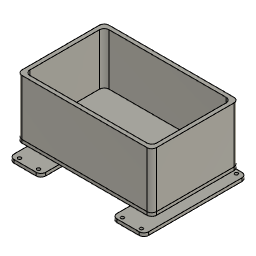
PondPumpFixture v5 (Autodesk Fusion 360 design; units mm, degrees)
Autodesk Fusion 360 part; units mm, degrees
sketch "Sketch1" plane through (0, 0, 0) normal (0, 0, 1) x (1, 0, 0)
  line L0 (0, 0) -> (160, 0)
  line L1 (160, 0) -> (160, 100)
  line L2 (160, 100) -> (0, 100)
  line L3 (0, 100) -> (0, 0)
  line L4 (0, 50) -> (160, 50) construction
  line L5 (125, 100) -> (125, 0) construction
  circle A0 centre (125, 84.5) radius 2
  circle A1 centre (125, 15.5) radius 2
  circle A2 centre (15, 85) radius 8
  circle A3 centre (15, 85) radius 4.75
  line L6 (-5, -5) -> (165, -5)
  line L7 (165, -5) -> (165, 105)
  line L8 (165, 105) -> (-5, 105)
  line L9 (-5, 105) -> (-5, -5)
  circle A4 centre (15, 15) radius 8
  circle A5 centre (15, 15) radius 4.75
  circle A6 centre (145, 85) radius 8
  circle A7 centre (145, 85) radius 4.75
  circle A8 centre (145, 15) radius 8
  circle A9 centre (145, 15) radius 4.75
  line L10 (-5, 105) -> (35, 105)
  line L11 (35, 105) -> (35, 115)
  line L12 (35, 115) -> (-5, 115)
  line L13 (-5, 115) -> (-5, 105)
  line L14 (15, 115) -> (15, -15) construction
  line L15 (-5, -5) -> (35, -5)
  line L16 (35, -5) -> (35, -15)
  line L17 (35, -15) -> (-5, -15)
  line L18 (-5, -15) -> (-5, -5)
  line L19 (-5, 110) -> (35, 110) construction
  circle A10 centre (3, 110) radius 2
  circle A11 centre (27, 110) radius 2
  line L20 (-5, -10) -> (35, -10) construction
  circle A12 centre (3, -10) radius 2
  circle A13 centre (27, -10) radius 2
  line L21 (35, -5) -> (35, 105)
  line L22 (165, 105) -> (125, 105)
  line L23 (125, 105) -> (125, 115)
  line L24 (125, 115) -> (165, 115)
  line L25 (165, 115) -> (165, 105)
  line L26 (165, -5) -> (125, -5)
  line L27 (125, -5) -> (125, -15)
  line L28 (125, -15) -> (165, -15)
  line L29 (165, -15) -> (165, -5)
  line L30 (125, -5) -> (125, 105)
  line L31 (145, 115) -> (145, -15) construction
  line L32 (125, 110) -> (165, 110) construction
  line L33 (125, -10) -> (165, -10) construction
  circle A14 centre (133, 110) radius 2
  circle A15 centre (157, 110) radius 2
  circle A16 centre (133, -10) radius 2
  circle A17 centre (157, -10) radius 2
  dimension "d1" = 160
  dimension "d2" = 100
  dimension "d3" = 4
  dimension "d4" = 4
  dimension "d5" = 34.5
  dimension "d6" = 34.5
  dimension "d7" = 35
  dimension "d8" = 16
  dimension "d9" = 9.5
  dimension "d12" = 5
  dimension "d13" = 16
  dimension "d14" = 9.5
  dimension "d16" = 15
  dimension "d17" = 16
  dimension "d18" = 9.5
  dimension "d19" = 16
  dimension "d20" = 9.5
  dimension "d22" = 15
  dimension "d23" = 15
  dimension "d25" = 40
  dimension "d26" = 10
  dimension "d28" = 40
  dimension "d29" = 10
  dimension "d30" = 15
  dimension "d31" = 4
  dimension "d32" = 4
  dimension "d33" = 8
  dimension "d34" = 8
  dimension "d35" = 4
  dimension "d36" = 4
  dimension "d37" = 8
  dimension "d38" = 8
  dimension "d39" = 40
  dimension "d40" = 10
  dimension "d41" = 40
  dimension "d42" = 10
  dimension "d43" = 4
  dimension "d44" = 4
  dimension "d45" = 8
  dimension "d46" = 8
  dimension "d47" = 4
  dimension "d48" = 4
  dimension "d49" = 8
  dimension "d50" = 8
  constraint horizontal L0
  constraint vertical L1
  constraint horizontal L2
  constraint vertical L3
  constraint coincident L0.start L3.end
  constraint midpoint L3 L4.start
  constraint midpoint L1 L4.end
  constraint coincident L2 L5.start
  constraint coincident L0 L5.end
  constraint perpendicular L0 L5
  constraint coincident L5 A0.centre
  constraint coincident L5 A1.centre
  constraint concentric A2 A3
  constraint concentric A4 A5
  constraint concentric A6 A7
  constraint concentric A8 A9
  constraint horizontal L10
  constraint vertical L11
  constraint horizontal L12
  constraint vertical L13
  constraint midpoint L12 L14.start
  constraint perpendicular L6 L14
  constraint horizontal L15
  constraint vertical L16
  constraint horizontal L17
  constraint vertical L18
  constraint midpoint L14.end L17
  constraint coincident A4.centre L14
  constraint coincident A2.centre L14
  constraint midpoint L13 L19.start
  constraint midpoint L11 L19.end
  constraint coincident L19 A10.centre
  constraint coincident L19 A11.centre
  constraint midpoint L18 L20.start
  constraint midpoint L16 L20.end
  constraint coincident L20 A12.centre
  constraint coincident L20 A13.centre
  constraint horizontal L22
  constraint vertical L23
  constraint horizontal L24
  constraint vertical L25
  constraint horizontal L26
  constraint vertical L27
  constraint horizontal L28
  constraint vertical L29
  constraint midpoint L24 L31.start
  constraint midpoint L28 L31.end
  constraint coincident A6.centre L31
  constraint coincident A8.centre L31
  constraint midpoint L23 L32.start
  constraint midpoint L25 L32.end
  constraint midpoint L27 L33.start
  constraint midpoint L29 L33.end
  constraint coincident L32 A14.centre
  constraint coincident L32 A15.centre
  constraint coincident L33 A16.centre
  constraint coincident L33 A17.centre
  measures "d1" distance of L0.start L0.end
  measures "d2" distance of L0.start L2.end
  measures "d3" diameter of A0
  measures "d4" diameter of A1
  measures "d5" distance of L4 A0.centre
  measures "d6" distance of L4 A1.centre
  measures "d7" distance of L1 L5
  measures "d8" diameter of A2
  measures "d9" diameter of A3
  measures "d13" diameter of A4
  measures "d14" diameter of A5
  measures "d16" distance of L0 A4.centre
  measures "d17" diameter of A6
  measures "d18" diameter of A7
  measures "d19" diameter of A8
  measures "d20" diameter of A9
  measures "d22" distance of L0 A8.centre
  measures "d23" distance of L2 A6.centre
  measures "d25" distance of L8.end L10.end
  measures "d26" distance of L8.end L12.end
  measures "d28" distance of L6.start L15.end
  measures "d29" distance of L6.start L17.end
  measures "d30" distance of L2 A2.centre
  measures "d31" diameter of A10
  measures "d32" diameter of A11
  measures "d33" distance of L19.end A11.centre
  measures "d34" distance of L13 A10.centre
  measures "d35" diameter of A12
  measures "d36" diameter of A13
  measures "d37" distance of L20.start A12.centre
  measures "d38" distance of L20.end A13.centre
  measures "d39" distance of L7.end L22.end
  measures "d40" distance of L7.end L24.end
  measures "d41" distance of L6.end L26.end
  measures "d42" distance of L6.end L28.end
  measures "d43" diameter of A14
  measures "d44" diameter of A15
  measures "d45" distance of L32.start A14.centre
  measures "d46" distance of L32.end A15.centre
  measures "d47" diameter of A16
  measures "d48" diameter of A17
  measures "d49" distance of L33.start A16.centre
  measures "d50" distance of L33.end A17.centre
extrude "Extrude1" add sketch "Sketch1" along normal blind 5 contours L0 L2 L3 L21 | L0 L2 L3 L6 L8 L9 L10 L15 L21 | L0 L2 A0 A1 L21 L30 | L0 L6 L21 L30 | L0 L1 L2 A0 A1 L30 | L0 L1 L2 L6 L7 L8 L22 L26 L30 | L2 L8 L21 L30 | A2 | A3 | A4 | A5 | A6 | A7 | A8 | A9 makes body 1
extrude "Extrude2" add sketch "Sketch1" along normal blind 70 contours L0 L2 L3 L6 L8 L9 L10 L15 L21 | L0 L6 L21 L30 | L0 L1 L2 L6 L7 L8 L22 L26 L30 | L2 L8 L21 L30 bodies 1
extrude "Extrude3" add sketch "Sketch1" against normal blind 4 separate body contours L0 L2 L3 L21 | L0 L2 L3 L6 L8 L9 L10 L15 L21 | L0 L2 A0 A1 L21 L30 | L0 L6 L21 L30 | L0 L1 L2 A0 A1 L30 | L0 L1 L2 L6 L7 L8 L22 L26 L30 | L2 L8 L21 L30 | A1 L30 | A1 L30 | A0 L30 | A0 L30 makes body 2
extrude "Extrude4" add sketch "Sketch1" against normal blind 2 from surface at -2 contours A2 | A4 | A6 | A8 bodies 2
extrude "Extrude5" add sketch "Sketch1" against normal blind 4 from surface at -17 separate body contours L0 L2 L3 L21 | L0 L2 L3 L6 L8 L9 L10 L15 L21 | L0 L1 L2 A0 A1 L30 | L0 L1 L2 L6 L7 L8 L22 L26 L30 | L6 L15 L16 L17 L18 | L6 L26 L27 L28 L29 | A1 L30 | L8 L10 L11 L12 L13 | A0 L30 | L8 L22 L23 L24 L25 picked at (125.6397, 15.3122) picked at (125.6397, 84.3122) makes body 3 at (-0.9702, 38.7308, -17) makes body 4 at (129.0298, 38.7308, -17)
extrude "Extrude6" add sketch "Sketch1" against normal blind 2 from surface at -17 contours A2 | A4 | A6 | A8 bodies 3 4
fillet "Fillet1" radius 6 18 edges at (160, 100, 37.5) (0, 0, 37.5) (-5, -5, 35) (0, 100, 37.5) (160, 0, 37.5) (165, -5, 35) (-5, -5, -2) (-5, 105, -2) (165, -5, -2) (165, 105, -2) (-5, -15, -19) (35, -15, -19) (35, 115, -19) (-5, 115, -19) (125, -15, -19) (165, -15, -19) (165, 115, -19) (125, 115, -19) on bodies 1 2 3 4
fillet "Fillet2" radius 6 2 edges at (165, 105, 35) (-5, 105, 35) on bodies 1
thread "Thread1" "ISO Metric profile 4.0 M4x0.7 6H" major diameter 4.1095 minor diameter 3.332 pitch 0.7 angle 60 modelled right hand crest width 0.193 on face at (126.5943, 85.7076, 3.3333) crest through (126.666, 84.5, 0.175) on bodies 1
thread "Thread2" "ISO Metric profile 4.0 M4x0.7 6H" major diameter 4.1095 minor diameter 3.332 pitch 0.7 angle 60 modelled right hand crest width 0.193 on face at (126.5943, 16.7076, 1.6667) crest through (126.666, 15.5, 0.175) on bodies 1
equation "d5 = ( 69 / 2 ) * 1 mm"
equation "d6 = ( 69 / 2 ) * 1 mm"
named bodies: "Tub", "TubBase", "Mount2", "Mount1"
